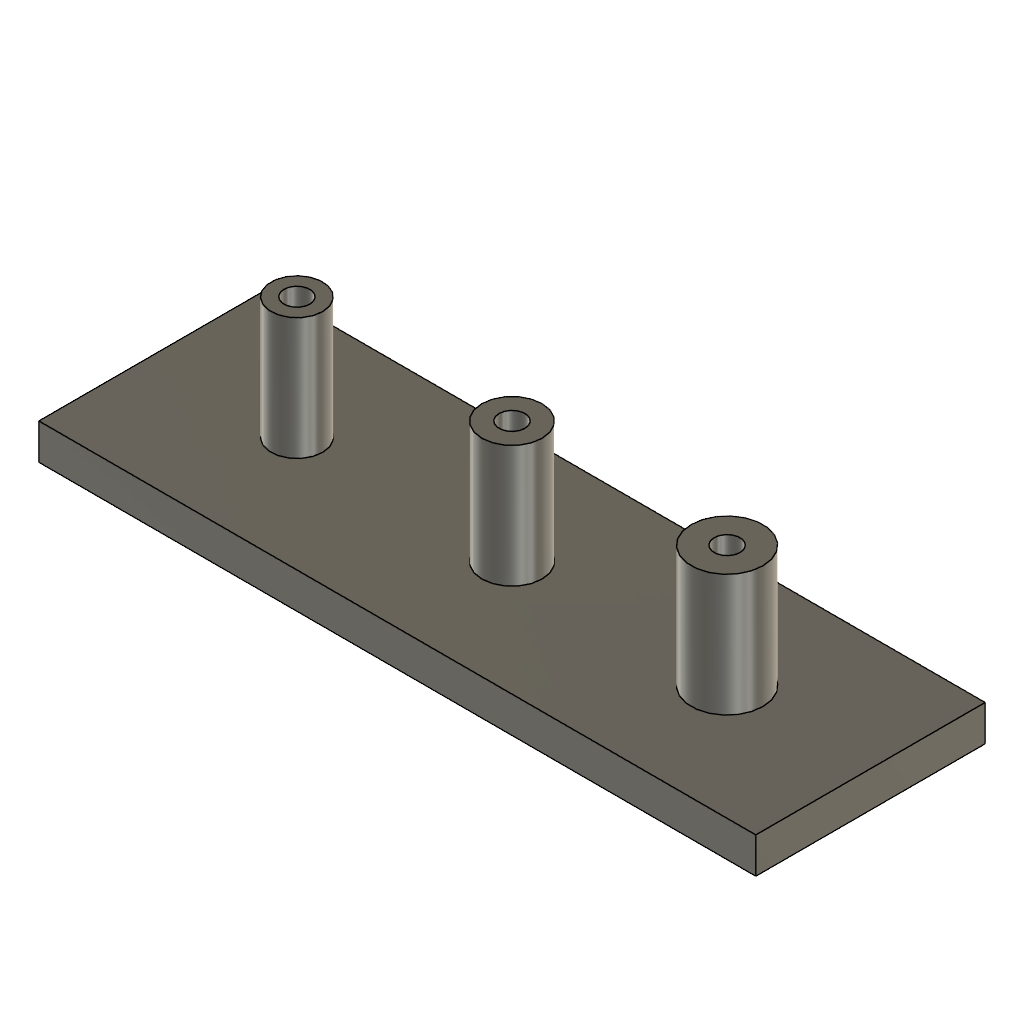
plaquette-plots (Autodesk Fusion 360 design; units mm, degrees)
part number: 2026-10-04-13-20-44-108
Autodesk Fusion 360 part; units mm, degrees
sketch "Esquisse1" plane through (0, 0, 0) normal (0, 0, 1) x (1, 0, 0)
  line L0 (0, 0) -> (50, 0)
  line L1 (50, 0) -> (50, 16)
  line L2 (50, 16) -> (0, 16)
  line L3 (0, 16) -> (0, 0)
  dimension "d7" = 50
  dimension "d8" = 16
  constraint horizontal L0
  constraint vertical L1
  constraint horizontal L2
  constraint vertical L3
  constraint coincident L0.start L3.end
  measures "d7" distance of L0.start L0.end
  measures "d8" distance of L0.start L2.end
extrude "Extrusion1" add sketch "Esquisse1" along normal blind 2.5
sketch "Esquisse2" plane through (0, 0, 2.5) normal (0, 0, 1) x (-1, 0, 0)
  line L0 (0, -16) -> (0, 0)
  line L1 (0, 0) -> (-50, 0)
  line L2 (-50, 0) -> (-50, -16)
  line L3 (-50, -16) -> (0, -16)
  circle A0 centre (-10, -8) radius 1.8
  dimension "d11" = 3.6
  dimension "d12" = 8
  dimension "d13" = 10
  measures "d11" diameter of A0
  measures "d12" distance of L3 A0.centre
  measures "d13" distance of L0 A0.centre
extrude "Extrusion2" add sketch "Esquisse2" along normal blind 8.5 contours A0
sketch "Esquisse3" plane through (0, 0, 2.5) normal (0, 0, 1) x (-1, 0, 0)
  circle A0 centre (-10, -8) radius 1.8
  line L0 (0, -16) -> (0, 0)
  line L1 (0, 0) -> (-50, 0)
  line L2 (-50, 0) -> (-50, -16)
  line L3 (-50, -16) -> (0, -16)
  circle A1 centre (-25, -8) radius 2.1
  dimension "d16" = 4.2
  dimension "d17" = 8
  dimension "d18" = 25
  measures "d16" diameter of A1
  measures "d17" distance of L3 A1.centre
  measures "d18" distance of L0 A1.centre
extrude "Extrusion3" add sketch "Esquisse3" along normal blind 8.5 contours A1
sketch "Esquisse4" plane through (0, 0, 2.5) normal (0, 0, 1) x (-1, 0, 0)
  circle A0 centre (-25, -8) radius 2.1
  circle A1 centre (-10, -8) radius 1.8
  line L0 (0, -16) -> (0, 0)
  line L1 (0, 0) -> (-50, 0)
  line L2 (-50, 0) -> (-50, -16)
  line L3 (-50, -16) -> (0, -16)
  circle A2 centre (-40, -8) radius 2.5
  dimension "d21" = 5
  dimension "d22" = 8
  dimension "d23" = 40
  measures "d21" diameter of A2
  measures "d22" distance of L3 A2.centre
  measures "d23" distance of L0 A2.centre
extrude "Extrusion4" add sketch "Esquisse4" along normal blind 8.5 contours A2
sketch "Esquisse5" plane through (0, 0, 11) normal (0, 0, 1) x (-1, 0, 0)
  circle A0 centre (-10, -8) radius 1.8
  circle A1 centre (-10, -8) radius 0.9
  dimension "d26" = 1.8
  constraint concentric A0 A1
  measures "d26" diameter of A1
extrude "Extrusion5" cut sketch "Esquisse5" against normal blind 6 contours A1
pattern_linear "Réseau R1" count 3 spacing 15 along (1, 0, 0) of "Extrusion5"
equation "l_plaque = 50 mm"
equation "w_plaque = 16 mm"
equation "ep_plaque = 2.5 mm"
equation "h_plot = 8.5 mm"
equation "d_pilote = 1.8 mm"
equation "p_pilote = 6 mm"
equation "d7 = l_plaque"
equation "d8 = w_plaque"
equation "d9 = ep_plaque"
equation "d14 = h_plot"
equation "d19 = h_plot"
equation "d24 = h_plot"
equation "d26 = d_pilote"
equation "d27 = -p_pilote"
